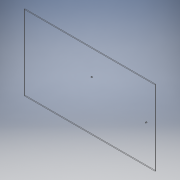
# Autodesk Inventor part: endplate
Saved by Autodesk Inventor 2018.2 (Build 222227000, 227)
## iProperties
Created: 2018-02-23
Part Number: endplate
Material: 一般
Document SubType Name: Modeling
Designer: ku_sk
Density: 1 g/cm^3
Appearance: 既定
Author: ku_sk
Autodesk Inventor part; units mm, degrees
ref_plane "YZ Plane" through (0, 0, 0) normal (1, 0, 0) x (0, 1, 0)
ref_plane "XZ Plane" through (0, 0, 0) normal (0, 1, 0) x (-1, 0, 0)
ref_plane "XY Plane" through (0, 0, 0) normal (0, 0, 1) x (1, 0, 0)
sketch "スケッチ1" plane through (0, 0, 0) normal (0, 1, 0) x (-1, 0, 0)
  line L0 (-350, 200) -> (350, 200)
  line L1 (350, 200) -> (350, -200)
  line L2 (350, -200) -> (-350, -200)
  line L3 (-350, -200) -> (-350, 200)
  line L4 (-350, 200) -> (350, -200) construction
  line L5 (350, 200) -> (-350, -200) construction
  point P0 (0, 0)
  dimension "d0" = 700
  dimension "d1" = 400
  constraints: 12 end point, 2 midpoint, 2 parallel, 1 horizontal, 1 perpendicular
  measures "d0" distance of L0.start L0.end
  measures "d1" distance of L2.end L0.start
extrude "押し出し1" add sketch "スケッチ1" along normal mid plane 5
sketch "スケッチ2" plane through (0, 2.5, 0) normal (0, 1, 0) x (1, 0, 0)
  circle A0 centre (300, 0) radius 2.5
  line L0 (-490, 0) -> (490, 0) projected
  point P0 (0, 0)
  dimension "d4" = 300
  dimension "d5" = 5
  constraints: 1 centre point, 1 point on line
  measures "d4" distance of point (0, 0) A0.centre
  measures "d5" diameter of A0
extrude "押し出し2" cut sketch "スケッチ2" against normal through all
sketch "スケッチ3" plane through (0, -2.5, 0) normal (0, -1, 0) x (1, 0, 0)
  circle A0 centre (20, 55) radius 2.5
  line L0 (350, -200) -> (350, 200) projected
  line L1 (-350, -200) -> (350, -200) projected
  point P0 (0, 0)
  dimension "d8" = 330
  dimension "d9" = 255
  dimension "d10" = 5
  constraints: 1 centre point
  measures "d8" distance from line of L0 A0.centre
  measures "d9" distance from line of L1 A0.centre
  measures "d10" diameter of A0
extrude "押し出し3" cut sketch "スケッチ3" against normal through all
